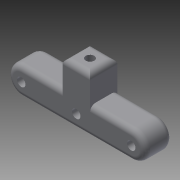
# Autodesk Inventor part: Part1
Saved by Autodesk Inventor 2015 (Build 190159000, 159)
## iProperties
Created: 2014-11-06
Part Number: Part1
Material: Generic
Document SubType Name: Modeling
Designer: ah14592
Density: 1 g/cm^3
Appearance: Default
Author: ah14592
Autodesk Inventor part; units mm, degrees
ref_plane "YZ Plane" through (0, 0, 0) normal (1, 0, 0) x (0, 1, 0)
ref_plane "XZ Plane" through (0, 0, 0) normal (0, 1, 0) x (-1, 0, 0)
ref_plane "XY Plane" through (0, 0, 0) normal (0, 0, 1) x (1, 0, 0)
sketch "Sketch1" plane through (0, 0, 0) normal (0, 1, 0) x (-1, 0, 0)
  arc A0 (0, -5) -> (0, 5) centre (0, 0) ccw
  arc A1 (-40, 5) -> (-40, -5) centre (-40, 0) ccw
  line L0 (0, 5) -> (-40, 5)
  line L1 (0, -5) -> (-40, -5)
  dimension "d2" = 40
  constraints: 4 end point, 4 point on circle, 2 centre point, 2 tangent, 1 coincident, 1 parallel
  measures "d2" distance of A1.centre point (0, 0)
extrude "Extrusion1" add sketch "Sketch1" along normal blind 10
sketch "Sketch2" plane through (0, 10, 0) normal (0, 1, 0) x (1, 0, 0)
  point P0 (0, 0)
hole "Hole1" at (0, 10, 0) direction (0, -1, 0) diameter 3.1 end through all counterbore diameter 4 counterbore depth 5
sketch "Sketch3" plane through (0, 10, 0) normal (0, 1, 0) x (1, 0, 0)
  arc A0 (40, -5) -> (40, 5) centre (40, 0) ccw projected
  point P0 (0, 0)
  point P1 (20, 0)
  constraints: 1 coincident
hole "Hole2" at (40, 10, 0) at (20, 10, 0) direction (0, -1, 0) diameter 3.1 end through all counterbore diameter 4 counterbore depth 5
sketch "Sketch4" plane through (0, 0, 5) normal (0, 0, 1) x (1, 0, 0)
  line L0 (21.55, 5) -> (18.45, 5) projected
  line L1 (40, 10) -> (0, 10) projected
  line L2 (40, 0) -> (0, 0) projected
  line L3 (15, 10) -> (25, 10)
  line L4 (25, 10) -> (25, 0)
  line L5 (25, 0) -> (15, 0)
  line L6 (15, 0) -> (15, 10)
  point P0 (20, 5)
  dimension "d19" = 10
  dimension "d20" = 5
  constraints: 8 end point, 2 parallel, 2 point on line, 1 horizontal, 1 midpoint, 1 perpendicular
  measures "d19" distance of L4.end L5.end
  measures "d20" distance from line of L6 point (20, 5)
extrude "Extrusion2" add sketch "Sketch4" along normal blind 10
fillet "Fillet1" radius 2 14 edges at (20, 10, 15) (15, 5, 15) (20, 0, 15) (25, 5, 15) (-5, 10, 0) (20, 10, -5) (45, 10, 0) (32.5, 10, 5) (7.5, 10, 5) (-5, 0, 0) (20, 0, -5) (45, 0, 0) (32.5, 0, 5) (7.5, 0, 5)
sketch "Sketch5" plane through (0, 0, 15) normal (0, 0, 1) x (1, 0, 0)
  line L0 (21.55, 5) -> (18.45, 5) projected
  point P0 (0, 0)
  point P1 (20, 5)
  constraints: 1 midpoint
hole "Hole3" at (20, 5, 15) direction (0, 0, -1) diameter 3.1 depth 8
body "Solid1"
